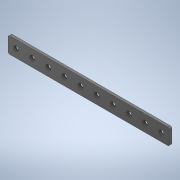
# Autodesk Inventor part: Noi nhom 20100
Saved by Autodesk Inventor 2020 (Build 240168000, 168)
## iProperties
Created: 2021-06-03
Part Number: Noi nhom 20100
Material: Generic
Document SubType Name: Modeling
Designer: admin
Density: 1 g/cm^3
Appearance: Smooth - Black
Author: admin
Autodesk Inventor part; units mm, degrees
ref_plane "YZ Plane" through (0, 0, 0) normal (1, 0, 0) x (0, 1, 0)
ref_plane "XZ Plane" through (0, 0, 0) normal (0, 1, 0) x (-1, 0, 0)
ref_plane "XY Plane" through (0, 0, 0) normal (0, 0, 1) x (1, 0, 0)
sketch "Sketch1" plane through (0, 0, 0) normal (0, 0, 1) x (1, 0, 0)
  line L0 (-100, -10) -> (100, -10)
  line L1 (100, -10) -> (100, 10)
  line L2 (100, 10) -> (-100, 10)
  line L3 (-100, 10) -> (-100, -10)
  line L4 (-100, -10) -> (100, 10) construction
  line L5 (100, -10) -> (-100, 10) construction
  point P0 (0, 0)
  dimension "d0" = 200
  dimension "d1" = 20
  constraints: 12 end point, 2 midpoint, 2 parallel, 1 horizontal, 1 perpendicular
  measures "d0" distance of L2.end L1.end
  measures "d1" distance of L1.end L0.end
extrude "Extrusion1" add sketch "Sketch1" along normal blind 3
sketch "Sketch2" plane through (0, 0, 3) normal (0, 0, 1) x (1, 0, 0)
  circle A0 centre (-90, 0) radius 3
  line L0 (-100, 10) -> (-100, -10) projected
  line L1 (100, 10) -> (-100, 10) projected
  point P0 (0, 0)
  dimension "d5" = 6
  dimension "d6" = 10
  dimension "d7" = 10
  constraints: 1 centre point
  measures "d5" diameter of A0
  measures "d6" distance from line of L0 A0.centre
  measures "d7" distance from line of L1 A0.centre
extrude "Extrusion2" cut sketch "Sketch2" against normal blind 3
pattern_linear "Rectangular Pattern1" count 10 spacing 20 along (1, 0, 0) of "Extrusion2"
fillet "Fillet1" radius 2 4 edges at (100, 10, 1.5) (100, -10, 1.5) (-100, -10, 1.5) (-100, 10, 1.5)
body "Solid1"
